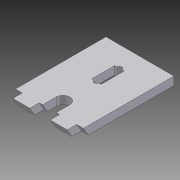
# Autodesk Inventor part: TRIANGLESHORTLEG
Saved by Autodesk Inventor 2012 SP2 (Build 160219200, 219)
## iProperties
Created: 2013-02-09
Part Number: TRIANGLESHORTLEG
Material: Default
Document SubType Name: Modeling
Designer: blacki
Density: 1 g/cm^3
Mass: 16.4659 g
Surface Area: 73.5691 cm^2
Volume: 16.4659 cm^3
Author: blacki
Autodesk Inventor part; units mm, degrees
ref_plane "YZ Plane" through (0, 0, 0) normal (1, 0, 0) x (0, 1, 0)
ref_plane "XZ Plane" through (0, 0, 0) normal (0, 1, 0) x (-1, 0, 0)
ref_plane "XY Plane" through (0, 0, 0) normal (0, 0, 1) x (1, 0, 0)
sketch "Sketch1" plane through (0, 0, 0) normal (0, 0, 1) x (1, 0, 0)
  line L0 (25, -30) -> (-25, -30)
  line L1 (-25, -30) -> (-25, 30)
  line L2 (-25, 30) -> (25, 30)
  line L3 (25, 30) -> (25, -30)
  line L4 (-25, 0) -> (25, 0) construction
  point P0 (0, 0)
  point P1 (0, 0)
  dimension "d0" = 50
  dimension "d1" = 60
  constraints: 10 end point, 3 midpoint, 2 parallel, 1 coincident, 1 horizontal, 1 perpendicular
  measures "d0" distance of L1.end L2.end
  measures "d1" distance of L0.end L1.end
extrude "Extrusion1" add sketch "Sketch1" along normal blind 6
sketch "Sketch2" plane through (-25, -30, 0) normal (-1, 0, 0) x (0, 0, 1)
  line L0 (0, 0) -> (6, 0) projected
  line L1 (6, -3.4641) -> (-173.2051, 100) construction
  line L2 (0, 0) -> (6, -3.4641)
  line L3 (6, -3.4641) -> (6, 0)
  point P0 (0, 30)
  constraints: 4 end point, 1 collinear, 1 perpendicular
extrude "Extrusion2" add sketch "Sketch2" against normal blind 50
sketch "Sketch4" plane through (-25, 30, 0) normal (-1, 0, 0) x (0, 0, 1)
  line L0 (6, -63.4641) -> (6, 0) projected
  line L1 (0, -60) -> (0, 0) projected
  line L2 (0, -60) -> (6, -63.4641) projected
  line L3 (6, -56.5359) -> (-167.2051, 43.4641) construction
  line L4 (0, -53.0718) -> (6, -56.5359)
  point P0 (0, -30)
  constraints: 2 end point, 2 point on line, 1 collinear
extrude "Extrusion3" cut sketch "Sketch4" against normal blind 5
sketch "Sketch7" plane through (0, 0, 0) normal (1, 0, 0) x (0, 1, 0)
  line L0 (-23.0718, 0) -> (-30, 0) construction
  line L1 (70, -173.2051) -> (-33.4641, 6) construction
  line L2 (-33.4641, 6) -> (-26.5359, 6) construction
  line L3 (-26.5359, 6) -> (73.4641, -167.2051) construction
  line L4 (-33.4641, 6) -> (-30, 0)
  line L5 (-23.0718, 0) -> (-30, 0)
  line L6 (-33.4641, 6) -> (-26.5359, 6)
  line L7 (-26.5359, 6) -> (-23.0718, 0)
  point P0 (0, 0)
  constraints: 8 end point, 2 collinear, 2 parallel
extrude "Extrusion6" cut sketch "Sketch7" along normal mid plane 15
mirror "Mirror1" about plane through (0, 0, 0) normal (1, 0, 0) of "Extrusion3"
sketch "Sketch8" plane through (0, 0, 6) normal (0, 0, 1) x (1, 0, 0)
  line L0 (-7.5, -26.5359) -> (7.5, -26.5359) projected
  line L1 (-5, -26.5359) -> (5, -26.5359)
  line L2 (5, -26.5359) -> (5, -16.5359)
  line L3 (5, -16.5359) -> (-5, -16.5359) construction
  line L4 (-5, -16.5359) -> (-5, -26.5359)
  arc A0 (5, -16.5359) -> (-5, -16.5359) centre (0, -16.5359) ccw
  point P0 (0, 0)
  point P1 (0, -26.5359)
  dimension "d23" = 10
  dimension "d24" = 10
  constraints: 8 end point, 3 midpoint, 2 parallel, 2 point on circle, 1 centre point, 1 horizontal, 1 perpendicular, 1 point on line
  measures "d23" distance of L3.end L2.end
  measures "d24" distance of L2.end L1.end
extrude "Extrusion7" cut sketch "Sketch8" against normal up to next
thicken "Thicken1" operation add thickness 10 both sides no extend neighbours yes toward (0, 1, 0) faces at (-8.3333, 30, 2)
sketch "Sketch11" plane through (0, 0, 6) normal (0, 0, 1) x (1, 0, 0)
  line L0 (-25, 40) -> (25, 40) projected
  line L1 (-3.5, 25) -> (3.5, 25)
  line L2 (3.5, 25) -> (3.5, 8)
  line L3 (3.5, 8) -> (-3.5, 8)
  line L4 (-3.5, 8) -> (-3.5, 25)
  line L5 (0, 40) -> (0, 0) construction
  line L6 (0, 40) -> (0, 0) construction
  circle A0 centre (0, 25) radius 1.75
  circle A1 centre (0, 8) radius 1.75
  dimension "d40" = 7
  dimension "d41" = 17
  dimension "d42" = 15
  dimension "d43" = 3.5
  dimension "d44" = 3.5
  constraints: 12 end point, 3 midpoint, 3 parallel, 2 centre point, 2 point on line, 1 coincident, 1 collinear, 1 horizontal, 1 perpendicular
  measures "d40" distance of L2.end L3.end
  measures "d41" distance of L1.end L2.end
  measures "d42" distance between parallel lines of L0 L1
  measures "d43" diameter of A0
  measures "d44" diameter of A1
extrude "Extrusion10" cut sketch "Sketch11" against normal up to next
equation "\"d44\" = d43"
body "Solid1"
